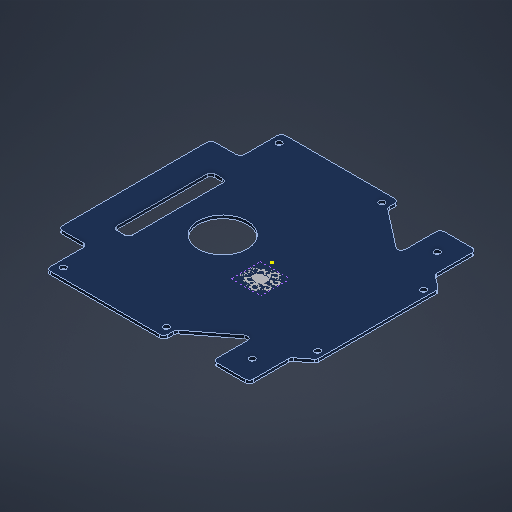
# Autodesk Inventor part: PCB
Saved by Autodesk Inventor 2026.1 (Build 301233020, 233B)
## iProperties
Created: 2026-02-13
Part Number: PCB
Material: Genérico
Document SubType Name: Modeling
Designer: celio
Density: 1 g/cm^3
Appearance: Padrão
Author: celio
Autodesk Inventor part; units mm, degrees
ref_plane "YZ Plane" through (0, 0, 0) normal (1, 0, 0) x (0, 1, 0)
ref_plane "XZ Plane" through (0, 0, 0) normal (0, 1, 0) x (-1, 0, 0)
ref_plane "XY Plane" through (0, 0, 0) normal (0, 0, 1) x (1, 0, 0)
sketch "Esboço1" plane through (0, 0, 0) normal (0, 1, 0) x (-1, 0, 0)
  line L0 (-70, 60) -> (70, 60)
  line L1 (70, 60) -> (70, -60)
  line L2 (70, -60) -> (-70, -60)
  line L3 (-70, -60) -> (-70, 60)
  line L4 (-70, 60) -> (70, -60) construction
  line L5 (70, 60) -> (-70, -60) construction
  point P0 (0, 0)
  dimension "d0" = 140
  dimension "d1" = 120
  constraints: 12 end point, 2 midpoint, 2 parallel, 1 horizontal, 1 perpendicular
  measures "d0" distance of L1.end L2.end
  measures "d1" distance of L0.end L1.end
extrude "Extrusão1" add sketch "Esboço1" along normal blind 1.6
sketch "Esboço2" plane through (0, 1.6, 0) normal (0, 1, 0) x (1, 0, 0)
  line L0 (-94.6357, 0) -> (83.6022, 0)
  line L1 (-70, -37) -> (-52, -37)
  line L2 (-52, 37) -> (-70, 37)
  line L3 (-70, 37) -> (-70, -37)
  line L4 (-70, -37) -> (-52, 37) construction
  line L5 (-52, -37) -> (-70, 37) construction
  line L6 (-70, 60) -> (-70, -60) projected
  line L7 (-70, 0) -> (-70, 0)
  line L8 (-70, 0) -> (-25, 0)
  circle A0 centre (-25, 0) radius 12.5
  line L9 (-70, -60) -> (70, -60) projected
  line L10 (-20, -60) -> (-50, -60)
  line L11 (-20, -60) -> (10, -60)
  line L12 (70, 60) -> (-70, 60) projected
  line L13 (-55, -60) -> (5, -60)
  line L14 (5, -60) -> (5, -45)
  line L15 (-55, -45) -> (-55, -60)
  line L16 (-52, 0) -> (-70, 0)
  line L17 (-56, 25) -> (-48, 25)
  line L18 (-48, 25) -> (-48, -25)
  line L19 (-48, -25) -> (-56, -25)
  line L20 (-56, -25) -> (-56, 25)
  line L21 (-56, 25) -> (-48, -25) construction
  line L22 (-48, 25) -> (-56, -25) construction
  line L23 (-55, 60) -> (5, 60)
  line L24 (5, 60) -> (5, 45)
  line L25 (-55, 45) -> (-55, 60)
  line L26 (-25, 76.0053) -> (-25, -77.5323)
  line L27 (-35, -45) -> (-35, -37)
  line L28 (-35, -37) -> (-15, -37)
  line L29 (-15, -37) -> (-15, -45)
  line L30 (5, -45) -> (-15, -45)
  line L31 (-35, -45) -> (-55, -45)
  line L32 (-35, 45) -> (-35, 37)
  line L33 (-35, 37) -> (-15, 37)
  line L34 (-15, 37) -> (-15, 45)
  line L35 (5, 45) -> (-15, 45)
  line L36 (-35, 45) -> (-55, 45)
  line L37 (-55, -60) -> (5, -45) construction
  line L38 (5, -60) -> (-55, -45) construction
  line L39 (-35, 45) -> (-15, 37) construction
  line L40 (-15, 45) -> (-35, 37) construction
  point P0 (0, 0)
  point P1 (-61, 0)
  point P2 (-25, 41)
  dimension "d4" = 18
  dimension "d5" = 74
  dimension "d6" = 0
  dimension "d7" = 45
  dimension "d8" = 25
  dimension "d28" = 15
  dimension "d30" = 18
  dimension "d31" = 8
  dimension "d32" = 50
  dimension "d35" = 15
  dimension "d36" = 20
  dimension "d38" = 8
  dimension "d40" = 20
  dimension "d41" = 8
  dimension "d42" = 60
  dimension "d43" = 60
  constraints: 76 end point, 11 parallel, 7 midpoint, 7 point on line, 6 perpendicular, 5 horizontal, 2 collinear, 2 vertical, 1 centre point, 1 coincident
  measures "d4" distance of L2.end L2.start
  measures "d5" distance of L2.start L1.end
  measures "d6" distance of L7.start L7.end
  measures "d7" distance of L7.start L8.end
  measures "d8" diameter of A0
  measures "d28" distance of L14.end L13.end
  measures "d30" distance of L16.start L7.start
  measures "d31" distance of L18.end L19.end
  measures "d32" distance of L17.end L18.end
  measures "d35" distance of L23.end L24.end
  measures "d36" distance of L27.end L28.end
  measures "d38" distance of L28.end L29.end
  measures "d40" distance of L32.end L33.end
  measures "d41" distance of L33.end L34.end
  measures "d42" distance of L13.start L13.end
  measures "d43" distance of L23.start L23.end
extrude "Extrusão4" cut sketch "Esboço2" against normal through all contours L26 A0 L0 | L26 A0 L0 | L0 A0 L26 | L0 A0 L26 | L18 L19 L20 L0 | L0 L20 L17 L18
sketch "Esboço3" plane through (0, 1.6, 0) normal (0, 1, 0) x (1, 0, 0)
  line L0 (44.5, -40) -> (30, -40) construction
  line L1 (30, -40) -> (30, -72.5) construction
  line L2 (30, -72.5) -> (44.5, -72.5) construction
  line L3 (44.5, -72.5) -> (44.5, -40) construction
  line L4 (30, 40) -> (44.5, 40) construction
  line L5 (44.5, 40) -> (44.5, 72.5) construction
  line L6 (44.5, 72.5) -> (30, 72.5) construction
  line L7 (30, 72.5) -> (30, 40) construction
  line L8 (37.25, -40) -> (37.25, -47.2) construction
  circle A0 centre (37.25, -47.2) radius 1.5
  line L9 (37.25, 40) -> (37.25, 47.2) construction
  circle A1 centre (37.25, 47.2) radius 1.5
  line L10 (-70, 60) -> (-70, -60) projected
  line L11 (52, 14) -> (49.5, 14) construction
  line L12 (49.5, 14) -> (49.5, -14) construction
  line L13 (49.5, -14) -> (52, -14) construction
  line L14 (52, -14) -> (52, 14) construction
  line L15 (52, 14) -> (49.5, -14) construction
  line L16 (49.5, 14) -> (52, -14) construction
  line L17 (54, 16) -> (47.5, 16)
  line L18 (47.5, 16) -> (47.5, -16) construction
  line L19 (47.5, -16) -> (54, -16) construction
  line L20 (54, -16) -> (54, 16)
  line L21 (70, -60) -> (70, 60) projected
  line L22 (5, -54.0532) -> (28, -36.1915)
  line L23 (28, -36.1915) -> (28, -58)
  line L24 (44.5, -69.5) -> (44.5446, -69.5)
  line L25 (46.5, -58) -> (46.5, -38)
  line L26 (46.5, -38) -> (46.5, -36.8245)
  line L27 (46.5, -58) -> (28, -58)
  line L28 (-70, -60) -> (70, -60) projected
  line L29 (7, -60) -> (5, -60)
  line L30 (70, 60) -> (-70, 60) projected
  line L31 (70, 60) -> (7, 60)
  line L32 (5, 54.0532) -> (28, 36.1915)
  line L33 (28, 58) -> (28, 36.1915)
  line L34 (44.5446, 69.5) -> (44.5, 69.5)
  line L35 (46.5, 58) -> (28, 58)
  line L36 (46.5, 36.8245) -> (46.5, 58)
  line L37 (5, 54.0532) -> (5, 60)
  line L38 (5, -54.0532) -> (5, -60)
  line L39 (54, -16) -> (54, -31)
  line L40 (54, -31) -> (46.5, -36.8245)
  line L41 (54, 16) -> (54, 31)
  line L42 (54, 31) -> (46.5, 36.8245)
  point P0 (0, 0)
  dimension "d59" = 14.5
  dimension "d60" = 32.5
  dimension "d63" = 32.5
  dimension "d64" = 14.5
  dimension "d76" = 7.2
  dimension "d77" = 3
  dimension "d78" = 7.2
  dimension "d79" = 3
  dimension "d97" = 2.5
  dimension "d98" = 28
  dimension "d99" = 2
  dimension "d103" = 2
  dimension "d104" = 2
  dimension "d105" = 63
  dimension "d107" = 2
  dimension "d132" = 15
  dimension "d133" = 15
  constraints: 78 end point, 10 parallel, 7 point on line, 6 perpendicular, 5 vertical, 3 horizontal, 2 centre point, 2 coincident, 2 midpoint, 3 other
  measures "d59" distance of L2.end L1.end
  measures "d60" distance of L1.end L0.end
  measures "d63" distance of L5.end L4.end
  measures "d64" distance of L5.end L6.end
  measures "d76" distance of L8.start L8.end
  measures "d77" diameter of A0
  measures "d78" distance of L9.start L9.end
  measures "d79" diameter of A1
  measures "d97" distance of L13.end L12.end
  measures "d98" distance of L12.end L11.end
  measures "d99" distance between parallel lines of L14 L20
  measures "d103" distance between parallel lines of L3 L25
  measures "d104" distance of L29.start L29.end
  measures "d105" distance of L21.end L31.end
  measures "d107" distance between parallel lines of L7 L33
  measures "d132" distance of L19.end L39.end
  measures "d133" distance of L17.start L41.end
sketch "Esboço4" plane through (0, 1.6, 0) normal (0, 1, 0) x (1, 0, 0)
  line L0 (-70, 60) -> (-70, -60) projected
  line L1 (-70, 0) -> (-70, -100)
  line L2 (-70, -100) -> (180, -100)
  line L3 (180, -100) -> (180, 100)
  line L4 (180, 100) -> (-70, 100)
  line L5 (-70, 100) -> (-70, -100)
  line L6 (250, 0) -> (-150, 0)
  line L7 (-430, 10) -> (570, 10)
  line L8 (570, 10) -> (570, -10)
  line L9 (570, -10) -> (-430, -10)
  line L10 (-430, -10) -> (-430, 10)
  line L11 (70, -60) -> (70, 60) projected
  line L12 (-430, 10) -> (570, -10) construction
  line L13 (570, 10) -> (-430, -10) construction
  line L14 (27.5, -90) -> (47.5, -90)
  line L15 (47.5, -90) -> (47.5, -50)
  line L16 (47.5, -50) -> (27.5, -50)
  line L17 (27.5, -50) -> (27.5, -90)
  line L18 (27.5, -90) -> (47.5, -50) construction
  line L19 (47.5, -90) -> (27.5, -50) construction
  line L20 (70, 60) -> (-70, 60) projected
  line L21 (47.5, 90) -> (27.5, 90)
  line L22 (27.5, 90) -> (27.5, 50)
  line L23 (27.5, 50) -> (47.5, 50)
  line L24 (47.5, 50) -> (47.5, 90)
  line L25 (47.5, 90) -> (27.5, 50) construction
  line L26 (27.5, 90) -> (47.5, 50) construction
  line L27 (0, -100) -> (0, 100) construction
  point P0 (0, 0)
  point P1 (70, 0)
  point P2 (37.5, -70)
  point P3 (37.5, 70)
  dimension "d53" = 100
  dimension "d54" = 250
  dimension "d55" = 200
  dimension "d65" = 1000
  dimension "d66" = 20
  dimension "d68" = 20
  dimension "d69" = 40
  dimension "d70" = 20
  dimension "d71" = 40
  dimension "d72" = 40
  dimension "d73" = 40
  dimension "d80" = 37.5
  dimension "d81" = 37.5
  constraints: 50 end point, 8 parallel, 6 midpoint, 5 horizontal, 5 perpendicular, 2 point on line, 1 collinear, 1 vertical
  measures "d53" distance of L1.start L1.end
  measures "d54" distance of L4.end L3.end
  measures "d55" distance of L3.end L2.end
  measures "d65" distance of L8.end L9.end
  measures "d66" distance of L7.end L8.end
  measures "d68" distance of L16.end L15.end
  measures "d69" distance of L15.end L14.end
  measures "d70" distance of L23.end L22.end
  measures "d71" distance of L22.end L21.end
  measures "d72" distance between parallel lines of L9 L16
  measures "d73" distance between parallel lines of L23 L7
  measures "d80" distance from line of L27 point (37.5, -70)
  measures "d81" distance from line of L27 point (37.5, 70)
extrude "Extrusão5" cut sketch "Esboço3" against normal through all contours A0 | A1
sketch "Esboço5" plane through (0, 1.6, 0) normal (0, 1, 0) x (1, 0, 0)
  line L0 (70, 60) -> (-70, 60) projected
  line L1 (-70, 60) -> (-55, 60)
  line L2 (-55, 60) -> (-55, 39)
  line L3 (-55, 39) -> (-70, 39)
  line L4 (-70, 39) -> (-70, 60)
  line L5 (-70, -60) -> (70, -60) projected
  line L6 (-70, -60) -> (-55, -60)
  line L7 (-55, -60) -> (-55, -39)
  line L8 (-55, -39) -> (-70, -39)
  line L9 (-70, -39) -> (-70, -60)
  line L10 (-70, 60) -> (-70, -60) projected
  line L11 (-55, 39) -> (-70, 39)
  line L12 (-70, 39) -> (-70, 60)
  line L13 (-70, 60) -> (-55, 60)
  line L14 (-55, 60) -> (-55, 39)
  line L15 (-55, -39) -> (-70, -39)
  line L16 (-70, -39) -> (-70, -60)
  line L17 (-70, -60) -> (-55, -60)
  line L18 (-55, -60) -> (-55, -39)
  point P0 (0, 0)
  dimension "d84" = 15
  dimension "d85" = 21
  dimension "d86" = 15
  dimension "d87" = 21
  constraints: 32 end point, 8 parallel, 4 horizontal, 4 perpendicular
  measures "d84" distance of L2.end L3.end
  measures "d85" distance of L1.end L2.end
  measures "d86" distance of L8.end L7.end
  measures "d87" distance of L7.end L6.end
extrude "Extrusão6" cut sketch "Esboço5" against normal through all
fillet "Arredondamento1" radius 2 10 edges at (-70, 0.8, 39) (-55, 0.8, 39) (-55, 0.8, 60) (-56, 0.8, 25) (-48, 0.8, 25) (-56, 0.8, -25) (-48, 0.8, -25) (-70, 0.8, -39) (-55, 0.8, -39) (-55, 0.8, -60)
sketch "Esboço7" plane through (0, 1.6, 0) normal (0, 1, 0) x (1, 0, 0)
  line L0 (-3.4695, -17.196) -> (-3.4695, -2.1961) construction
  line L1 (-3.4695, -2.1961) -> (11.6526, -2.1961) construction
  line L2 (11.6526, -2.1961) -> (11.6526, -17.196) construction
  line L3 (11.6526, -17.196) -> (-3.4695, -17.196) construction
  point P0 (0, 0)
  constraints: 2 other
extrude "Extrusão10" cut sketch "Esboço3" against normal through all contours L30 L21 L28 L38 L22 L23 L27 L25 L26 L40 L39 L20 L41 L42 L36 L35 L33 L32 L37
fillet "Arredondamento4" radius 2 14 edges at (5, 0.8, 60) (5, 0.8, 54.0532) (28, 0.8, 36.1915) (28, 0.8, 58) (46.5, 0.8, 58) (46.5, 0.8, 36.8245) (54, 0.8, 31) (54, 0.8, -31) (46.5, 0.8, -36.8245) (46.5, 0.8, -58) (28, 0.8, -58) (28, 0.8, -36.1915) (5, 0.8, -54.0532) (5, 0.8, -60)
sketch "Esboço8" plane through (0, 1.6, 0) normal (0, 1, 0) x (1, 0, 0)
  line L0 (-55, -60) -> (5, -60)
  line L1 (5, -60) -> (5, -50)
  line L2 (5, -50) -> (-55, -50)
  line L3 (-55, -50) -> (-55, -60)
  circle A0 centre (-51.25, -55) radius 1.5
  circle A1 centre (1.25, -55) radius 1.5
  line L4 (-70, 37) -> (-70, -37) projected
  line L5 (-70, 0) -> (54, 0)
  line L6 (54, 30.0209) -> (54, -30.0209) projected
  line L7 (-55, 60) -> (5, 60)
  line L8 (5, 60) -> (5, 50)
  line L9 (5, 50) -> (-55, 50)
  line L10 (-55, 50) -> (-55, 60)
  circle A2 centre (-51.25, 55) radius 1.5
  circle A3 centre (1.25, 55) radius 1.5
  point P0 (0, 0)
  point P1 (-55, -55)
  dimension "d137" = 60
  dimension "d138" = 10
  dimension "d140" = 3
  dimension "d142" = 3
  dimension "d143" = 3.75
  dimension "d144" = 3.75
  dimension "d145" = 5
  dimension "d146" = 5
  dimension "d147" = 60
  dimension "d148" = 10
  dimension "d149" = 3
  dimension "d150" = 3
  dimension "d151" = 3.75
  dimension "d152" = 5
  dimension "d153" = 5
  dimension "d154" = 3.75
  constraints: 18 end point, 4 centre point, 4 parallel, 3 midpoint, 2 horizontal, 2 perpendicular
  measures "d137" distance of L2.end L1.end
  measures "d138" distance of L1.end L0.end
  measures "d140" diameter of A0
  measures "d142" diameter of A1
  measures "d143" distance from line of L1 A1.centre
  measures "d144" distance of point (-55, -55) A0.centre
  measures "d145" distance from line of L0 A0.centre
  measures "d146" distance from line of L0 A1.centre
  measures "d147" distance of L8.end L9.end
  measures "d148" distance of L7.end L8.end
  measures "d149" diameter of A2
  measures "d150" diameter of A3
  measures "d151" distance from line of L10 A2.centre
  measures "d152" distance from line of L7 A2.centre
  measures "d153" distance from line of L7 A3.centre
  measures "d154" distance from line of L8 A3.centre
extrude "Extrusão11" cut sketch "Esboço8" against normal through all contours A0 | A1 | A2 | A3
sketch "Esboço9" plane through (0, 1.6, 0) normal (0, 1, 0) x (1, 0, 0)
  line L0 (54, -38.06) -> (50.5, -38.06)
  line L1 (50.5, -38.06) -> (50.5, 41.775)
  line L2 (50.5, 41.775) -> (54, 41.775)
  line L3 (54, 41.775) -> (54, -38.06)
  line L4 (52.2999, -27) -> (48.7001, -27)
  line L5 (48.7001, -27) -> (48.7001, 27)
  line L6 (48.7001, 27) -> (52.2999, 27)
  line L7 (52.2999, 27) -> (52.2999, -27)
  line L8 (52.2999, -27) -> (48.7001, 27) construction
  line L9 (48.7001, -27) -> (52.2999, 27) construction
  circle A0 centre (50.5, -27) radius 1.5
  circle A1 centre (50.5, 27) radius 1.5
  point P0 (0, 0)
  point P1 (50.5, 0)
  dimension "d158" = 3.5
  dimension "d159" = 54
  dimension "d160" = 3
  dimension "d161" = 3
  constraints: 20 end point, 4 midpoint, 4 parallel, 2 centre point, 2 horizontal, 2 perpendicular, 1 point on line
  measures "d158" distance of L1.end L2.end
  measures "d159" distance of L4.end L5.end
  measures "d160" diameter of A0
  measures "d161" diameter of A1
extrude "Extrusão12" cut sketch "Esboço9" against normal through all contours A0 L4 L1 | L1 L4 A0 | L4 A0 L1 | L1 A0 L4 | A1 L6 L1 | L1 L6 A1 | L6 A1 L1 | L1 A1 L6
